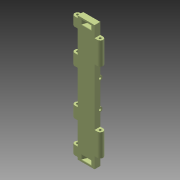
# Autodesk Inventor part: 载板
Saved by Autodesk Inventor 2015 (Build 190159000, 159)
## iProperties
Created: 2017-05-02
Part Number: 载板
Material: 常规
Document SubType Name: Modeling
Designer: Administrator
Density: 1 g/cm^3
Appearance: 铬酸锌 2
Author: Administrator
Autodesk Inventor part; units mm, degrees
ref_plane "YZ Plane" through (0, 0, 0) normal (1, 0, 0) x (0, 1, 0)
ref_plane "XZ Plane" through (0, 0, 0) normal (0, 1, 0) x (-1, 0, 0)
sketch "草图1" plane through (0, 0, 0) normal (0, 0, 1) x (1, 0, 0)
  line L0 (-75, 25) -> (0, 25)
  line L1 (0, 25) -> (0, 0)
  line L2 (0, 0) -> (-75, 0)
  line L3 (-75, 0) -> (-75, 25)
  dimension "d0" = 75
  dimension "d1" = 25
  constraints: 8 end point, 2 parallel, 1 horizontal, 1 perpendicular
  measures "d0" distance of L0.start L0.end
  measures "d1" distance of L2.end L0.start
extrude "拉伸1" add sketch "草图1" against normal blind 550
sketch "草图2" plane through (-75, 25, 0) normal (0, 1, 0) x (1, 0, 0)
  line L0 (15, 35) -> (65, 35)
  line L1 (65, 35) -> (65, 515)
  line L2 (65, 515) -> (15, 515)
  line L3 (15, 515) -> (15, 35)
  line L4 (0, 0) -> (0, 550) projected
  point P0 (75, 0)
  dimension "d4" = 480
  dimension "d5" = 50
  dimension "d6" = 15
  dimension "d7" = 35
  constraints: 8 end point, 2 parallel, 1 horizontal, 1 perpendicular
  measures "d4" distance of L2.end L0.start
  measures "d5" distance of L0.start L0.end
  measures "d6" distance between parallel lines of L4 L3
  measures "d7" distance from line of point (75, 0) L0
extrude "拉伸2" cut sketch "草图2" against normal blind 20
sketch "草图3" plane through (0, 0, 0) normal (1, 0, 0) x (0, 0, -1)
  line L0 (35, 25) -> (35, 5) projected
  line L1 (35, 14.9983) -> (45, 5)
  line L2 (35, 5) -> (515, 5) projected
  point P0 (0, 0)
  dimension "d10" = 134.995
  dimension "d11" = 10
  constraints: 2 end point, 2 point on line
  measures "d10" angle of L0 L1
  measures "d11" distance of L0.end L1.end
extrude "拉伸3" add sketch "草图3" against normal blind 60
pattern_linear "矩形阵列1" count 8 spacing 60 along (0, 0, -1) of "拉伸3"
sketch "草图4" plane through (0, 0, 0) normal (1, 0, 0) x (0, 0, -1)
  line L0 (515, 25) -> (515, 5) projected
  line L1 (515, 15) -> (505, 5)
  line L2 (515, 5) -> (465, 5) projected
  line L3 (505, 5) -> (515, 5)
  point P0 (0, 0)
  dimension "d17" = 45
  dimension "d18" = 10
  constraints: 4 end point, 1 horizontal, 1 midpoint, 1 point on line
  measures "d17" angle of L0 L1
  measures "d18" distance of L1.end L0.end
extrude "拉伸4" add sketch "草图4" against normal blind 60
pattern_linear "矩形阵列2" count 8 spacing 60 along (0, 0, 1) of "拉伸4"
sketch "草图5" plane through (0, 0, 0) normal (1, 0, 0) x (0, 0, -1)
  line L0 (35, 25) -> (515, 25) projected
  arc A0 (105, 25) -> (85, 25) centre (95, 25) ccw
  line L1 (0, 25) -> (550, 25) projected
  point P0 (0, 0)
  dimension "d24" = 95
  dimension "d25" = 10
  constraints: 3 point on line, 2 point on circle, 1 centre point
  measures "d24" horizontal distance of point (0, 0) A0.centre
  measures "d25" radius of A0
extrude "拉伸5" add sketch "草图5" against normal blind 70
sketch "草图6" plane through (0, 0, 0) normal (1, 0, 0) x (0, 0, -1)
  circle A0 centre (95, 25) radius 5
  arc A1 (105, 25) -> (85, 25) centre (95, 25) ccw projected
  point P0 (0, 0)
  dimension "d28" = 10
  constraints: 1 centre point, 1 concentric
  measures "d28" diameter of A0
extrude "拉伸6" cut sketch "草图6" against normal blind 70
pattern_linear "矩形阵列3" count 4 spacing 120 along (0, 0, -1) of "拉伸5", "拉伸6"
sketch "草图7" plane through (0, 0, 0) normal (0, 0, 1) x (1, 0, 0)
  line L0 (-60, 25) -> (-10, 25)
  line L1 (-10, 25) -> (-10, 35)
  line L2 (-10, 35) -> (-60, 35)
  line L3 (-60, 35) -> (-60, 25)
  line L4 (-60, 25) -> (-60, 14.9983) projected
  line L5 (-10, 25) -> (-10, 14.9983) projected
  point P0 (0, 0)
  dimension "d34" = 10
  constraints: 8 end point, 2 collinear, 2 parallel, 1 horizontal, 1 perpendicular
  measures "d34" distance of L2.end L0.start
extrude "拉伸7" cut sketch "草图7" against normal blind 550
sketch "草图8" plane through (-75, 0, 0) normal (-1, 0, 0) x (0, 0, 1)
  line L0 (0, 25) -> (-550, 25) projected
  line L1 (-110, 25) -> (-80, 25)
  line L2 (-80, 25) -> (-80, 5)
  line L3 (-80, 5) -> (-110, 5)
  line L4 (-110, 5) -> (-110, 25)
  line L5 (0, 0) -> (-550, 0) projected
  dimension "d37" = 30
  dimension "d38" = 80
  dimension "d39" = 5
  constraints: 8 end point, 2 parallel, 1 horizontal, 1 perpendicular, 1 point on line
  measures "d37" distance of L2.end L3.end
  measures "d38" distance from line of L5.start L2
  measures "d39" distance between parallel lines of L5 L3
extrude "拉伸8" cut sketch "草图8" against normal blind 5
sketch "草图9" plane through (-70, 0, 0) normal (-1, 0, 0) x (0, 0, 1)
  circle A0 centre (-105, 20) radius 1.5
  circle A1 centre (-102, 10) radius 1.5
  circle A2 centre (-88, 10) radius 1.5
  circle A3 centre (-85, 20) radius 1.5
  line L0 (-80, 25) -> (-80, 5) projected
  line L1 (-110, 5) -> (-110, 25) projected
  line L2 (-85, 25) -> (-80, 25) projected
  line L3 (-110, 25) -> (-105, 25) projected
  line L4 (-80, 5) -> (-110, 5) projected
  point P0 (0, 0)
  dimension "d42" = 3
  dimension "d43" = 3
  dimension "d44" = 3
  dimension "d45" = 3
  dimension "d46" = 8
  dimension "d47" = 8
  dimension "d48" = 5
  dimension "d49" = 5
  dimension "d50" = 5
  dimension "d51" = 5
  dimension "d52" = 5
  dimension "d53" = 5
  constraints: 4 centre point
  measures "d42" diameter of A0
  measures "d43" diameter of A1
  measures "d44" diameter of A2
  measures "d45" diameter of A3
  measures "d46" distance from line of L0 A2.centre
  measures "d47" distance from line of L1 A1.centre
  measures "d48" distance from line of L0 A3.centre
  measures "d49" distance from line of L1 A0.centre
  measures "d50" distance from line of L2 A3.centre
  measures "d51" distance from line of L3 A0.centre
  measures "d52" distance from line of L4 A2.centre
  measures "d53" distance from line of L4 A1.centre
extrude "拉伸9" cut sketch "草图9" against normal blind 10
thread "螺纹1" size "M3x0.5" class "6H" standard "ANSI Metric M Profile" full length
thread "螺纹2" size "M3x0.5" class "6H" standard "ANSI Metric M Profile" full length
thread "螺纹3" size "M3x0.5" class "6H" standard "ANSI Metric M Profile" full length
thread "螺纹4" size "M3x0.5" class "6H" standard "ANSI Metric M Profile" full length
pattern_linear "矩形阵列4" count 4 spacing 120 along (0, 0, -1) of "拉伸8", "拉伸9"
sketch "草图10" plane through (0, 0, 0) normal (0, 0, 1) x (1, 0, 0)
  arc A0 (-87.5, 25) -> (-87.5, 0) centre (-87.5, 12.5) ccw
  arc A1 (12.5, 0) -> (12.5, 25) centre (12.5, 12.5) ccw
  line L0 (-75, 0) -> (0, 0) projected
  line L1 (-75, 25) -> (-75, 0) projected
  line L2 (0, 0) -> (0, 25) projected
  line L3 (-87.5, 25) -> (-75, 25)
  line L4 (-87.5, 0) -> (-75, 0)
  line L5 (12.5, 25) -> (0, 25)
  line L6 (12.5, 0) -> (0, 0)
  circle A2 centre (-87.5, 12.5) radius 5
  circle A3 centre (12.5, 12.5) radius 5
  line L7 (-75, 25) -> (-75, 0)
  line L8 (0, 25) -> (0, 0)
  dimension "d67" = 25
  dimension "d68" = 25
  dimension "d69" = 10
  dimension "d70" = 10
  constraints: 12 end point, 5 tangent, 4 centre point, 4 point on circle, 2 coincident, 2 point on line, 2 vertical, 1 parallel
  measures "d67" diameter of A0
  measures "d68" diameter of A1
  measures "d69" diameter of A2
  measures "d70" diameter of A3
extrude "拉伸10" add sketch "草图10" against normal blind 550
sketch "草图11" plane through (-87.5, 25, -550) normal (0, 1, 0) x (1, 0, 0)
  line L0 (12.5, -500) -> (-12.5, -500)
  line L1 (-12.5, -500) -> (-12.5, -400)
  line L2 (-12.5, -400) -> (12.5, -400)
  line L3 (12.5, -400) -> (12.5, -500)
  line L4 (12.5, -470) -> (12.5, -440) projected
  line L5 (100, -550) -> (0, -550) projected
  line L6 (12.5, -350) -> (-12.5, -350)
  line L7 (-12.5, -350) -> (-12.5, -200)
  line L8 (-12.5, -200) -> (12.5, -200)
  line L9 (12.5, -200) -> (12.5, -350)
  line L10 (-12.5, -550) -> (-12.5, 0) projected
  line L11 (12.5, -50) -> (-12.5, -50)
  line L12 (-12.5, -50) -> (-12.5, -150)
  line L13 (-12.5, -150) -> (12.5, -150)
  line L14 (12.5, -150) -> (12.5, -50)
  line L15 (0, 0) -> (100, 0) projected
  line L16 (112.5, -550) -> (112.5, 0) projected
  line L17 (87.5, -50) -> (112.5, -50)
  line L18 (112.5, -50) -> (112.5, 0)
  line L19 (112.5, 0) -> (87.5, 0)
  line L20 (87.5, 0) -> (87.5, -50)
  line L21 (87.5, -150) -> (112.5, -150)
  line L22 (112.5, -150) -> (112.5, -200)
  line L23 (87.5, -400) -> (87.5, -150)
  line L24 (112.5, -150) -> (112.5, -400)
  line L25 (112.5, -400) -> (87.5, -400)
  line L26 (87.5, -400) -> (87.5, -350)
  line L27 (87.5, -500) -> (112.5, -500)
  line L28 (112.5, -500) -> (112.5, -550)
  line L29 (112.5, -550) -> (87.5, -550)
  line L30 (87.5, -550) -> (87.5, -500)
  line L31 (87.5, -100) -> (87.5, -90) projected
  dimension "d73" = 25
  dimension "d74" = 100
  dimension "d75" = 150
  dimension "d76" = 50
  dimension "d77" = 50
  dimension "d78" = 100
  dimension "d79" = 50
  constraints: 52 end point, 12 parallel, 9 collinear, 8 point on line, 6 horizontal, 6 perpendicular
  measures "d73" distance of L1.end L2.end
  measures "d74" distance of L0.end L1.end
  measures "d75" distance between parallel lines of L5 L2
  measures "d76" distance between parallel lines of L2 L6
  measures "d77" distance between parallel lines of L15 L11
  measures "d78" distance of L13.end L11.start
  measures "d79" distance between parallel lines of L8 L13
extrude "拉伸11" cut sketch "草图11" against normal blind 25
ref_plane "工作平面1" through (0, 0, -10) normal (0, 0, 1) x (1, 0, 0)
sketch "草图12" plane through (0, 0, -10) normal (0, 0, 1) x (1, 0, 0)
  line L0 (-16.0581, 0) -> (-56.0581, 0)
  line L1 (-56.0581, 0) -> (-46.0581, 25)
  line L2 (-46.0581, 25) -> (-26.0581, 25)
  line L3 (-26.0581, 25) -> (-16.0581, 0)
  line L4 (-36.0581, 0) -> (-36.0581, -9.5048)
  line L5 (-87.5, 0) -> (0, 0) projected
  line L6 (0, 25) -> (-87.5, 25) projected
  point P0 (-36.0581, 25)
  dimension "d83" = 40
  dimension "d84" = 20
  constraints: 10 end point, 2 collinear, 2 midpoint, 1 horizontal, 1 parallel, 1 point on line, 1 vertical
  measures "d83" distance of L0.start L0.end
  measures "d84" distance of L1.end L2.end
extrude "拉伸12" cut sketch "草图12" against normal blind 15
fillet "圆角1" radius 6 4 edges at (-16.0581, 0, -17.5) (-56.0581, 0, -17.5) (-46.0581, 25, -17.5) (-26.0581, 25, -17.5)
fillet "圆角2" radius 4 12 edges at (-14.027, 0, -10) (-36.0581, 0, -10) (-58.0892, 0, -10) (-14.027, 0, -25) (-36.0581, 0, -25) (-58.0892, 0, -25) (-50.4892, 25, -25) (-36.0581, 25, -25) (-21.627, 25, -25) (-50.4892, 25, -10) (-36.0581, 25, -10) (-21.627, 25, -10)
pattern_linear "矩形阵列5" count 2 spacing 515 along (0, 0, -1) of "拉伸12", "圆角1", "圆角2"
sketch "草图13" plane through (-60, 25, -35) normal (0, 1, 0) x (1, 0, 0)
  line L0 (-15, -35) -> (-40, -35)
  line L1 (-40, -35) -> (-40, -25)
  line L2 (-40, -25) -> (-15, -25)
  line L3 (-15, -25) -> (-15, -35)
  line L4 (-15, 45) -> (-15, 15) projected
  line L5 (37.1472, -25) -> (10.7365, -25) projected
  line L6 (-15, 505) -> (-40, 505)
  line L7 (-40, 505) -> (-40, 515)
  line L8 (-40, 515) -> (-15, 515)
  line L9 (-15, 515) -> (-15, 505)
  line L10 (-15, 465) -> (-15, 435) projected
  line L11 (-27.5, 515) -> (60, 515) projected
  point P0 (60, -35)
  dimension "d92" = 10
  dimension "d93" = 25
  dimension "d94" = 10
  dimension "d95" = 25
  constraints: 16 end point, 4 collinear, 4 parallel, 2 horizontal, 2 perpendicular
  measures "d92" distance of L0.end L1.end
  measures "d93" distance of L0.start L0.end
  measures "d94" distance of L6.end L7.end
  measures "d95" distance of L7.end L8.end
extrude "拉伸13" cut sketch "草图13" against normal blind 25
